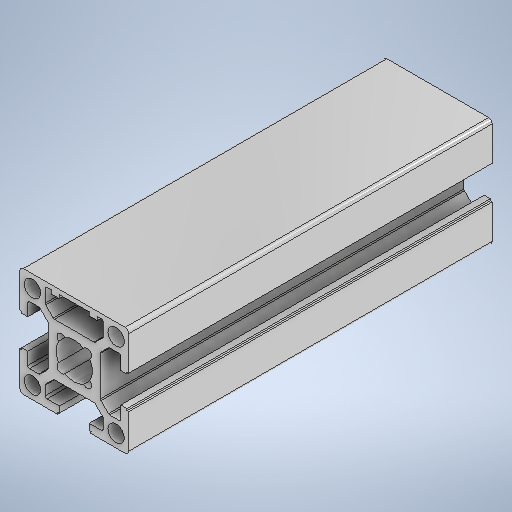
# Autodesk Inventor part: Perfil 30×30 3 rasgos_001
Saved by Autodesk Inventor 2026 (Build 300175000, 175)
## iProperties
Created: 2025-04-05
Part Number: Perfil 30×30 3 rasgos_001
Material: Aluminum 6061
Document SubType Name: Modeling
Designer: Tony Dias
Density: 2.7 g/cm^3
Appearance: Aluminum - Polished
Author: Tony Dias
Autodesk Inventor part; units mm, degrees
sketch "Sketch1" plane through (0, 0, 0) normal (0, 0, 1) x (1, 0, 0)
  circle A0 centre (0, 0) radius 5 construction
  line L0 (-15, 15) -> (0, 0) construction
  circle A1 centre (-3.5355, 3.5355) radius 1.25 construction
  circle A2 centre (-3.5355, -3.5355) radius 1.25 construction
  circle A3 centre (3.5355, -3.5355) radius 1.25 construction
  circle A4 centre (3.5355, 3.5355) radius 1.25 construction
  line L1 (-7.2, 7.2) -> (0, 7.2) construction
  line L2 (-7.2, 7.2) -> (-7.2, 0) construction
  line L3 (-15, -15) -> (0, 0) construction
  line L4 (-9.5556, 8) -> (-7.2, 5.6444)
  circle A5 centre (-11.5, 11.5) radius 2.25
  line L5 (-15, 15) -> (-15, 4.1) construction
  line L6 (-15, 4.1) -> (-14.5, 4.1) construction
  line L7 (-14.5, 4.1) -> (-14.5, 4.6)
  line L8 (-14.5, 4.6) -> (-15, 4.6)
  line L9 (-15, 4.6) -> (-15, 4.1) construction
  line L10 (-15, 15) -> (-15, 4.6)
  line L11 (-12.8, 8) -> (-12.8, 4.1)
  line L12 (-12.8, 8) -> (-9.5556, 8)
  line L13 (-7.2, 5.6444) -> (-7.2, 0)
  line L14 (-8, 9.5556) -> (-5.6444, 7.2)
  line L15 (-8, 15) -> (-8, 8) construction
  line L16 (-15, 15) -> (0, 15)
  line L17 (-8, 13.75) -> (-8, 9.5556)
  line L18 (-8, 13.75) -> (-6.3, 13.75)
  line L19 (-6.3, 13.75) -> (-6.3, 12.8)
  line L20 (-6.3, 12.8) -> (-4.1, 12.8)
  line L21 (-4.1, 12.8) -> (-4.1, 13.75)
  line L22 (-4.1, 13.75) -> (0, 13.75)
  line L23 (0, 15) -> (0, 13.75)
  line L24 (-7.2, 0) -> (-7.2, -5.6444)
  line L25 (-15, 0) -> (0, 0) construction
  line L26 (-7.2, -5.6444) -> (-9.5556, -8)
  line L27 (-12.8, -8) -> (-9.5556, -8)
  line L28 (-12.8, -4.1) -> (-12.8, -8)
  line L29 (-15, 4.1) -> (-12.8, 4.1) construction
  line L30 (-14.5, 4.1) -> (-12.8, 4.1)
  circle A6 centre (-11.5, -11.5) radius 2.25
  line L31 (-15, -4.1) -> (-12.8, -4.1) construction
  line L32 (-15, -4.1) -> (-14.5, -4.1) construction
  line L33 (-14.5, -4.1) -> (-14.5, -4.6)
  line L34 (-14.5, -4.6) -> (-15, -4.6)
  line L35 (-15, -4.6) -> (-15, -4.1) construction
  line L36 (-14.5, -4.1) -> (-12.8, -4.1)
  line L37 (-15, -15) -> (-15, -4.6)
  line L38 (-15, -15) -> (-4.1, -15) construction
  line L39 (-4.1, -15) -> (-4.6, -15) construction
  line L40 (-4.6, -15) -> (-4.6, -14.5)
  line L41 (-4.6, -14.5) -> (-4.1, -14.5)
  line L42 (-4.1, -14.5) -> (-4.1, -15) construction
  line L43 (-15, -15) -> (-4.6, -15)
  line L44 (-4.1, -15) -> (-4.1, -12.8) construction
  line L45 (-4.1, -12.8) -> (-4.1, -14.5)
  line L46 (-8, -12.8) -> (-4.1, -12.8)
  line L47 (-8, -9.5556) -> (-8, -12.8)
  line L48 (-5.6444, -7.2) -> (-8, -9.5556)
  line L49 (-5.6444, -7.2) -> (0, -7.2)
  line L50 (-5.6444, 7.2) -> (0, 7.2)
  arc A7 (-2.5481, -4.302) -> (0, -5) centre (0, 0) ccw
  arc A8 (-4.302, -2.5481) -> (-2.5481, -4.302) centre (-3.5355, -3.5355) ccw
  arc A9 (-5, 0) -> (-4.302, -2.5481) centre (0, 0) ccw
  arc A10 (-4.302, 2.5481) -> (-5, 0) centre (0, 0) ccw
  arc A11 (-2.5481, 4.302) -> (-4.302, 2.5481) centre (-3.5355, 3.5355) ccw
  arc A12 (0, 5) -> (-2.5481, 4.302) centre (0, 0) ccw
  line L51 (0, 7.2) -> (0, 5)
  line L52 (0, -5) -> (0, -7.2)
  point P0 (0, 7.2)
  dimension "d0" = 10
  dimension "d1" = 15
  dimension "d2" = 15
  dimension "d3" = 2.5
  dimension "d6" = 360
  dimension "d8" = 2.2
  dimension "d9" = 15
  dimension "d10" = 15
  dimension "d12" = 4.5
  dimension "d13" = 11.5
  dimension "d14" = 11.5
  dimension "d15" = 1.1
  dimension "d16" = 4.1
  dimension "d17" = 0.5
  dimension "d19" = 1.25
  dimension "d20" = 1.25
  dimension "d22" = 2.2
  dimension "d23" = 4.1
  dimension "d24" = 2.2
  dimension "d25" = 4.1
  constraints: 106 end point, 18 horizontal, 17 vertical, 16 point on circle, 14 equal length, 12 centre point, 8 parallel, 8 point on line, 8 vertical alignment, 4 coincident, 4 perpendicular, 3 horizontal alignment, 2 concentric, 1 collinear, 1 equal radius, 26 other
  measures "d1" horizontal distance of point (0, 0) L0.start
  measures "d2" horizontal distance of point (0, 0) L0.start
  measures "d3" diameter of A1
  measures "d9" horizontal distance of point (0, 0) L3.start
  measures "d10" horizontal distance of point (0, 0) L3.start
  measures "d12" diameter of A5
  measures "d13" horizontal distance of point (0, 0) A5.centre
  measures "d14" horizontal distance of A5.centre point (0, 0)
  measures "d15" distance between parallel lines of L0 L4
  measures "d16" vertical distance of point (0, 0) L5.end
  measures "d17" distance of L7.end L8.end
  measures "d19" distance edge to line of A5 L12
  measures "d20" distance from line of L16 L17.start
  measures "d22" distance between parallel lines of L16 L20
  measures "d23" horizontal distance of point (0, 0) L20.end
  measures "d24" distance of L5.end L11.end
  measures "d25" horizontal distance of point (0, 0) L38.end
extrude "Extrusion1" add sketch "Sketch1" along normal mid plane 100
mirror "Mirror1" about plane through (0, 0, 0) normal (1, 0, 0) of "Extrusion1"
fillet "Fillet1" radius 1 4 edges at (15, 15, 0) (15, -15, 0) (-15, 15, 0) (-15, -15, 0)
fillet "Fillet2" radius 0.5 24 edges at (-12.8, -8, 0) (-9.5556, -8, 0) (-8, -12.8, 0) (9.5556, -8, 0) (7.2, -5.6444, 0) (5.6444, 7.2, 0) (-5.6444, 7.2, 0) (-8, 9.5556, 0) (-7.2, 5.6444, 0) (-7.2, -5.6444, 0) (8, -12.8, 0) (8, -9.5556, 0) (12.8, -8, 0) (8, 9.5556, 0) (8, 13.75, 0) (9.5556, 8, 0) (12.8, 8, 0) (-9.5556, 8, 0) (-8, 13.75, 0) (-12.8, 8, 0) (-5.6444, -7.2, 0) (-8, -9.5556, 0) (5.6444, -7.2, 0) (7.2, 5.6444, 0)
equation "\"d1\" = d2"
equation "\"d9\" = d2"
equation "\"d10\" = d2"
equation "\"d14\" = d13"
equation "\"d20\" = d19"
equation "\"d23\" = d16"
equation "\"d25\" = d16"
body "Solid1"
